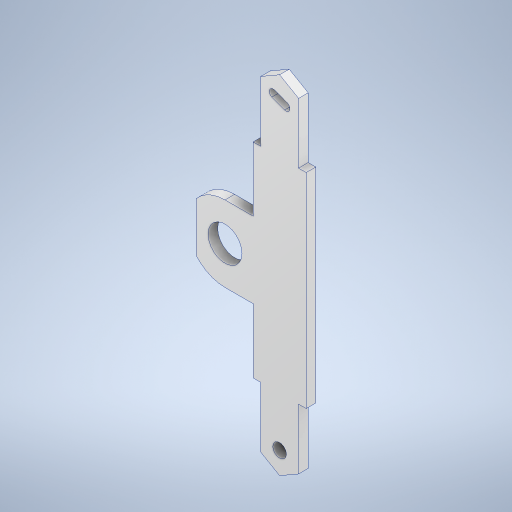
# Autodesk Inventor part: Z-Axis Nut and Bed Plate
Saved by Autodesk Inventor 2024 (Build 280153000, 153)
## iProperties
Created: 2024-08-02
Part Number: Z-Axis Nut and Bed Plate
Material: Aluminum 6061
Document SubType Name: Modeling
Designer: Ishaan
Density: 2.7 g/cm^3
Appearance: Aluminum - Flat
Author: Ishaan
Autodesk Inventor part; units mm, degrees
ref_plane "YZ Plane" through (0, 0, 0) normal (1, 0, 0) x (0, 1, 0)
ref_plane "XZ Plane" through (0, 0, 0) normal (0, 1, 0) x (-1, 0, 0)
ref_plane "XY Plane" through (0, 0, 0) normal (0, 0, 1) x (1, 0, 0)
sketch "Sketch1" plane through (0, 0, 0) normal (0, 0, 1) x (1, 0, 0)
  line L0 (12.5, -107.2169) -> (-12.5, -107.2169)
  line L1 (-12.5, -107.2169) -> (-12.5, 107.2169)
  line L2 (-12.5, 107.2169) -> (12.5, 107.2169)
  line L3 (12.5, 107.2169) -> (12.5, -107.2169)
  line L4 (12.5, -107.2169) -> (-12.5, 107.2169) construction
  line L5 (-12.5, -107.2169) -> (12.5, 107.2169) construction
  line L6 (0, 100) -> (0, -100) construction
  line L7 (-12.5, 107.2169) -> (0, 114.4338)
  line L8 (0, 114.4338) -> (12.5, 107.2169)
  line L9 (12.5, 107.2169) -> (12.5, 92.7831)
  line L10 (12.5, 92.7831) -> (0, 85.5662)
  line L11 (0, 85.5662) -> (-12.5, 92.7831)
  line L12 (-12.5, 92.7831) -> (-12.5, 107.2169)
  line L13 (-12.5, -107.2169) -> (-12.5, -92.7831)
  line L14 (-12.5, -92.7831) -> (0, -85.5662)
  line L15 (0, -85.5662) -> (12.5, -92.7831)
  line L16 (12.5, -92.7831) -> (12.5, -107.2169)
  line L17 (12.5, -107.2169) -> (0, -114.4338)
  line L18 (0, -114.4338) -> (-12.5, -107.2169)
  line L19 (-4.2122, 101.5835) -> (4.2122, 98.4165) construction
  line L20 (-5.1447, 99.103) -> (3.2797, 95.936)
  line L21 (5.1447, 100.897) -> (-3.2797, 104.064)
  arc A0 (-3.2797, 104.064) -> (-5.1447, 99.103) centre (-4.2122, 101.5835) ccw
  arc A1 (3.2797, 95.936) -> (5.1447, 100.897) centre (4.2122, 98.4165) ccw
  circle A2 centre (0, -100) radius 4.5
  circle A3 centre (-36, 0) radius 11.2
  circle A4 centre (-36, 0) radius 21 construction
  line L22 (-21, -14.6969) -> (-51, -14.6969) construction
  line L23 (-51, -14.6969) -> (-51, 14.6969) construction
  line L24 (-51, 14.6969) -> (-21, 14.6969) construction
  line L25 (-21, 14.6969) -> (-21, -14.6969) construction
  line L26 (-21, -14.6969) -> (-51, 14.6969) construction
  line L27 (-51, -14.6969) -> (-21, 14.6969) construction
  circle A5 centre (-36, 0) radius 25
  line L28 (-55, 16.2481) -> (-55, -16.2481)
  line L29 (-12.5, 25) -> (-36, 25)
  line L30 (-36, 25) -> (-36, -25)
  line L31 (-36, -25) -> (-12.5, -25)
  line L32 (-12.5, -25) -> (-12.5, 25)
  line L33 (17.5, -67.375) -> (-17.5, -67.375)
  line L34 (-17.5, -67.375) -> (-17.5, 67.375)
  line L35 (-17.5, 67.375) -> (17.5, 67.375)
  line L36 (17.5, 67.375) -> (17.5, -67.375)
  line L37 (17.5, -67.375) -> (-17.5, 67.375) construction
  line L38 (-17.5, -67.375) -> (17.5, 67.375) construction
  point P0 (0, 0)
  point P1 (266, 0)
  point P2 (-17.5, -25)
  point P3 (-12.5, -67.375)
  point P4 (-12.5, 67.375)
  point P5 (-17.5, 25)
  point P6 (-36, 25)
  point P7 (12.5, 67.375)
  point P8 (12.5, -67.375)
  dimension "d8" = 42
  dimension "d0" = 25
  dimension "d1" = 266
  dimension "d2" = 200
  dimension "d3" = 5.3
  dimension "d4" = 9
  dimension "d5" = 9
  dimension "d6" = 22.4
  dimension "d7" = 36
  dimension "d9" = 30
  dimension "d10" = 4
  dimension "d11" = 4
  dimension "d12" = 134.75
  dimension "d13" = 35
  constraints: 80 end point, 9 parallel, 8 midpoint, 7 point on circle, 6 tangent, 5 centre point, 5 coincident, 5 perpendicular, 4 horizontal, 3 point on line, 2 collinear, 2 horizontal alignment, 1 vertical, 29 other
  measures "d0" distance of L2.end L1.end
  measures "d1" distance of point (266, 0) point (0, 0)
  measures "d2" distance of L6.start L6.end
  measures "d3" diameter of A1
  measures "d4" distance of L19.start L19.end
  measures "d5" diameter of A2
  measures "d6" diameter of A3
  measures "d7" distance of point (0, 0) A3.centre
  measures "d9" distance between parallel lines of L25 L23
  measures "d11" distance between parallel lines of L23 L28
  measures "d12" distance of L35.end L33.start
  measures "d13" distance between parallel lines of L36 L34
extrude "Extrusion1" add sketch "Sketch1" along normal blind 6.35 contours L17 L18 L0 | L0 L1 L14 L15 L3 | L15 L14 L1 L33 L3 | L33 L1 A5 L35 L3 | L3 L35 L36 L33 | L33 L34 L31 L1 | L35 L1 L11 L10 L3 | L31 L34 A5 L1 | L10 L11 L1 L2 L3 | L1 L29 L34 L35 | A5 L34 L1 | L1 A5 | L31 A5 L34 | L2 L7 L8 | L1 A5 L34 L29 | A5 L30 A3 L34 | A5 L28 L30 A3 | L34 A5 L29
sketch "Sketch2" plane through (0, 0, 6.35) normal (0, 0, 1) x (1, 0, 0)
  line L0 (-17.5, -25) -> (-17.5, -67.375) projected
  line L1 (-17.5, -67.375) -> (-12.5, -67.375) projected
  line L2 (-12.5, -67.375) -> (-12.5, -107.2169) projected
  line L3 (-12.5, -107.2169) -> (0, -114.4338) projected
  line L4 (0, -114.4338) -> (12.5, -107.2169) projected
  line L5 (12.5, -107.2169) -> (12.5, -67.375) projected
  line L6 (12.5, -67.375) -> (17.5, -67.375) projected
  line L7 (17.5, -67.375) -> (17.5, 67.375) projected
  line L8 (17.5, 67.375) -> (12.5, 67.375) projected
  line L9 (12.5, 67.375) -> (12.5, 107.2169) projected
  line L10 (12.5, 107.2169) -> (0, 114.4338) projected
  line L11 (0, 114.4338) -> (-12.5, 107.2169) projected
  line L12 (-12.5, 107.2169) -> (-12.5, 67.375) projected
  line L13 (-12.5, 67.375) -> (-17.5, 67.375) projected
  line L14 (-17.5, 67.375) -> (-17.5, 25) projected
  line L15 (-17.5, 25) -> (-36, 25) projected
  arc A0 (-36, 25) -> (-55, 16.2481) centre (-36, 0) ccw projected
  line L16 (-55, 16.2481) -> (-55, -16.2481) projected
  arc A1 (-55, -16.2481) -> (-36, -25) centre (-36, 0) ccw projected
  line L17 (-36, -25) -> (-17.5, -25) projected
  circle A2 centre (-36, 0) radius 11.2 projected
  arc A3 (-3.2797, 104.064) -> (-5.1447, 99.103) centre (-4.2122, 101.5835) ccw projected
  line L18 (-3.2797, 104.064) -> (5.1447, 100.897) projected
  arc A4 (3.2797, 95.936) -> (5.1447, 100.897) centre (4.2122, 98.4165) ccw projected
  line L19 (3.2797, 95.936) -> (-5.1447, 99.103) projected
  circle A5 centre (0, -100) radius 4.5 projected
  circle A6 centre (-13.25, 68.125) radius 1.375
  point P0 (0, 0)
  point P1 (-12.5, 69.2774)
  point P2 (-14.4024, 67.375)
  dimension "d16" = 0.75
  dimension "d17" = 2.75
  dimension "d18" = 0.75
  constraints: 1 centre point
  measures "d16" distance from line of L12 A6.centre
  measures "d17" diameter of A6
  measures "d18" distance from line of A6.centre L13
sketch "Sketch3" plane through (0, 0, 6.35) normal (0, 0, 1) x (1, 0, 0)
  circle A0 centre (0, -100) radius 4.5 projected
  arc A1 (-3.2797, 104.064) -> (-5.1447, 99.103) centre (-4.2122, 101.5835) ccw projected
  line L0 (-3.2797, 104.064) -> (5.1447, 100.897) projected
  arc A2 (3.2797, 95.936) -> (5.1447, 100.897) centre (4.2122, 98.4165) ccw projected
  line L1 (3.2797, 95.936) -> (-5.1447, 99.103) projected
  circle A3 centre (-36, 0) radius 11.2 projected
  arc A4 (14.4024, -67.375) -> (12.5, -69.2774) centre (13.25, -68.125) ccw projected
  line L2 (14.4024, -67.375) -> (17.5, -67.375) projected
  line L3 (17.5, -67.375) -> (17.5, 67.375) projected
  line L4 (17.5, 67.375) -> (14.4024, 67.375) projected
  arc A5 (12.5, 69.2774) -> (14.4024, 67.375) centre (13.25, 68.125) ccw projected
  line L5 (12.5, 69.2774) -> (12.5, 107.2169) projected
  line L6 (12.5, 107.2169) -> (0, 114.4338) projected
  line L7 (0, 114.4338) -> (-12.5, 107.2169) projected
  line L8 (-12.5, 107.2169) -> (-12.5, 69.2774) projected
  arc A6 (-14.4024, 67.375) -> (-12.5, 69.2774) centre (-13.25, 68.125) ccw projected
  line L9 (-14.4024, 67.375) -> (-17.5, 67.375) projected
  line L10 (-17.5, 67.375) -> (-17.5, 25) projected
  line L11 (-17.5, 25) -> (-36, 25) projected
  arc A7 (-36, 25) -> (-55, 16.2481) centre (-36, 0) ccw projected
  line L12 (-55, 16.2481) -> (-55, -16.2481) projected
  arc A8 (-55, -16.2481) -> (-36, -25) centre (-36, 0) ccw projected
  line L13 (-36, -25) -> (-17.5, -25) projected
  line L14 (-17.5, -25) -> (-17.5, -67.375) projected
  line L15 (-17.5, -67.375) -> (-14.4024, -67.375) projected
  arc A9 (-12.5, -69.2774) -> (-14.4024, -67.375) centre (-13.25, -68.125) ccw projected
  line L16 (-12.5, -69.2774) -> (-12.5, -107.2169) projected
  line L17 (-12.5, -107.2169) -> (0, -114.4338) projected
  line L18 (0, -114.4338) -> (12.5, -107.2169) projected
  line L19 (12.5, -107.2169) -> (12.5, -69.2774) projected
  circle A10 centre (-36, 0) radius 16 construction
  line L20 (-36, 0) -> (-24.6863, 11.3137) construction
  line L21 (-36, 0) -> (-36, 16) construction
  line L22 (-36, 0) -> (-36, -16) construction
  line L23 (-47.3137, -11.3137) -> (-24.6863, -11.3137) construction
  line L24 (-24.6863, -11.3137) -> (-24.6863, 11.3137) construction
  line L25 (-24.6863, 11.3137) -> (-47.3137, 11.3137) construction
  line L26 (-47.3137, 11.3137) -> (-47.3137, -11.3137) construction
  line L27 (-47.3137, -11.3137) -> (-24.6863, 11.3137) construction
  line L28 (-24.6863, -11.3137) -> (-47.3137, 11.3137) construction
  point P0 (0, 0)
  dimension "d21" = 32
  dimension "d22" = 45
  constraints: 18 end point, 7 coincident, 3 point on circle, 2 midpoint, 2 parallel, 1 centre point, 1 horizontal, 1 perpendicular, 1 point on line, 1 vertical
  measures "d21" diameter of A10
  measures "d22" angle of L20 L21
sketch "Sketch4" plane through (0, 0, 6.35) normal (0, 0, 1) x (1, 0, 0)
  line L0 (10, -57.375) -> (-10, -57.375) construction
  line L1 (-10, -57.375) -> (-10, 57.375) construction
  line L2 (-10, 57.375) -> (10, 57.375) construction
  line L3 (10, 57.375) -> (10, -57.375) construction
  line L4 (10, -57.375) -> (-10, 57.375) construction
  line L5 (-10, -57.375) -> (10, 57.375) construction
  line L6 (-17.5, -67.375) -> (-14.4024, -67.375) construction
  point P0 (0, 0)
  point P1 (-10, 0)
  point P2 (10, 0)
  dimension "d30" = 20
  dimension "d32" = 10
  constraints: 12 end point, 4 coincident, 4 midpoint, 2 parallel, 1 horizontal, 1 perpendicular
  measures "d30" distance of L1.end L2.end
  measures "d32" distance between parallel lines of L0 L6
equation "\"d11\" = d10"
equation "\"d18\" = d16"
body "Solid1"
